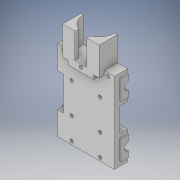
# Autodesk Inventor part: x 캐리지
Saved by Autodesk Inventor 2018 (Build 220112000, 112)
## iProperties
Created: 2019-01-22
Part Number: x 캐리지
Material: Generic
Document SubType Name: Modeling
Designer: User
Density: 1 g/cm^3
Appearance: Default
Author: User
Autodesk Inventor part; units mm, degrees
ref_plane "YZ Plane" through (0, 0, 0) normal (1, 0, 0) x (0, 1, 0)
ref_plane "XZ Plane" through (0, 0, 0) normal (0, 1, 0) x (-1, 0, 0)
ref_plane "XY Plane" through (0, 0, 0) normal (0, 0, 1) x (1, 0, 0)
sketch "스케치1" plane through (0, 0, 0) normal (1, 0, 0) x (0, 1, 0)
  arc A0 (33.25, -13) -> (18.25, -13) centre (25.75, -13) ccw
  arc A1 (-18.25, -13) -> (-33.25, -13) centre (-25.75, -13) ccw
  line L0 (-37.5, 0) -> (35.75, 0)
  line L1 (33.25, -13) -> (35.75, -13)
  line L2 (18.25, -13) -> (15.75, -13)
  line L3 (15.75, -13) -> (15.75, -5.5)
  line L4 (-18.25, -13) -> (-15.75, -13)
  line L5 (-15.75, -13) -> (-15.75, -5.5)
  line L6 (-33.25, -13) -> (-35.75, -13)
  line L7 (-35.75, -13) -> (-35.75, -5.5)
  line L8 (-15.75, -13) -> (-11.75, -13)
  line L9 (-11.75, -13) -> (-11.75, -5.5)
  line L10 (-35.75, -13) -> (-39.75, -13)
  line L11 (-39.75, -13) -> (-39.75, -5.5)
  line L12 (15.75, -13) -> (11.75, -13)
  line L13 (11.75, -13) -> (11.75, -5.5)
  line L14 (35.75, -13) -> (39.75, -13)
  line L15 (25.75, -5.5) -> (15.75, -5.5)
  line L16 (35.75, -5.5) -> (25.75, -5.5)
  line L17 (15.75, -5.5) -> (11.75, -5.5)
  line L18 (11.75, -5.5) -> (-11.75, -5.5)
  line L19 (-15.75, -5.5) -> (-25.75, -5.5)
  line L20 (-35.75, -5.5) -> (-25.75, -5.5)
  line L21 (-11.75, -5.5) -> (-15.75, -5.5)
  arc A2 (29.85, -13) -> (21.65, -13) centre (25.75, -13) ccw
  line L22 (33.25, -13) -> (29.85, -13)
  line L23 (21.65, -13) -> (18.25, -13)
  arc A3 (-21.65, -13) -> (-29.85, -13) centre (-25.75, -13) ccw
  line L24 (-18.25, -13) -> (-21.65, -13)
  line L25 (-29.85, -13) -> (-33.25, -13)
  line L26 (29.85, -13) -> (21.65, -13)
  line L27 (-21.65, -13) -> (-29.85, -13)
  line L28 (35.75, 2) -> (60.75, 2)
  line L29 (60.75, 2) -> (60.75, -13)
  line L30 (35.75, 2) -> (35.75, 0)
  line L31 (35.75, 2) -> (35.75, 5)
  line L32 (35.75, 5) -> (60.75, 5)
  line L33 (60.75, 5) -> (63.75, 5)
  line L34 (63.75, 5) -> (63.75, 2)
  line L35 (63.75, 2) -> (63.75, -13)
  line L36 (63.75, -13) -> (60.75, -13)
  line L37 (-37.5, 0) -> (-39.75, 0)
  line L38 (-39.75, 0) -> (-39.75, -5.5)
  line L39 (-35.75, -5.5) -> (-35.75, 0)
  line L40 (39.75, 0) -> (39.75, -13)
  line L41 (35.75, 0) -> (35.75, -5.5)
  line L42 (35.75, -13) -> (35.75, -5.5)
  line L43 (39.75, 0) -> (39.75, 2)
  line L44 (60.75, -13) -> (39.75, -13)
  line L45 (35.75, 5) -> (31.75, 5)
  line L46 (31.75, 5) -> (31.75, 0)
  line L47 (39.75, 0) -> (35.75, 0)
  point P0 (0, 0)
  dimension "d1" = 37.5
  dimension "d8" = 2.5
  dimension "d10" = 2.5
  dimension "d11" = 4
  dimension "d12" = 4
  dimension "d13" = 4
  dimension "d28" = 8.2
  dimension "d29" = 8.2
  dimension "d37" = 25
  dimension "d38" = 3
  dimension "d39" = 3
  dimension "d81" = 4
  constraints: 96 end point, 13 horizontal, 10 point on circle, 9 perpendicular, 9 point on line, 8 collinear, 4 centre point, 3 vertical, 2 coincident, 1 parallel, 1 tangent
  measures "d1" distance of point (0, 0) L0.start
  measures "d8" distance of L2.start L2.end
  measures "d10" distance of L6.start L6.end
  measures "d11" distance of L4.end L8.end
  measures "d12" distance of L6.end L10.end
  measures "d13" distance of L2.end L12.end
  measures "d28" diameter of A2
  measures "d29" diameter of A3
  measures "d37" distance of L28.start L28.end
  measures "d38" distance of L28.start L31.end
  measures "d39" distance of L32.end L33.end
  measures "d81" distance of L31.end L45.end
extrude "돌출1" add sketch "스케치1" along normal mid plane 56 contours L15 L17 L18 L21 L19 L20 L39 L0 L41 L16
extrude "돌출3" add sketch "스케치1" along normal mid plane 56 contours L3 L12 L13 L17 | L9 L8 L5 L21
extrude "돌출4" add sketch "스케치1" along normal mid plane 56 contours L15 L17 L18 L21 L19 L20 L39 L0 L41 L16 | L39 L7 L10 L11 L38 L37 L0
extrude "돌출5" add sketch "스케치1" along normal mid plane 52 contours A0 L16 L42 L1 | A0 L2 L3 L15 | L5 L4 A1 L19 | A1 L6 L7 L20
extrude "돌출6" add sketch "스케치1" along normal mid plane 3.8 contours L22 A2 L23 A0 | A1 L24 A3 L25
sketch "스케치3" plane through (26, 0, 0) normal (1, 0, 0) x (0, 0, -1)
  line L0 (5.5, 15.75) -> (5.5, 35.75) projected
  line L1 (13, 11.75) -> (13, 15.75) projected
  line L2 (5.5, 35.75) -> (13, 35.75)
  line L3 (13, 15.75) -> (5.5, 15.75)
  line L4 (5.5, 15.75) -> (5.5, 35.75)
  line L5 (13, 18.25) -> (13, 21.65) projected
  arc A0 (13, 29.85) -> (13, 21.65) centre (13, 25.75) ccw
  line L6 (13, 35.75) -> (13, 29.85)
  line L7 (13, 21.65) -> (13, 15.75)
  line L8 (5.5, -15.75) -> (13, -15.75) projected
  line L9 (13, -35.75) -> (13, -39.75) projected
  line L10 (5.5, -15.75) -> (13, -15.75)
  line L11 (13, -35.75) -> (5.5, -35.75)
  line L12 (5.5, -35.75) -> (5.5, -15.75)
  line L13 (13, -33.25) -> (13, -29.85) projected
  arc A1 (13, -21.65) -> (13, -29.85) centre (13, -25.75) ccw
  line L14 (13, -15.75) -> (13, -21.65)
  line L15 (13, -29.85) -> (13, -35.75)
  point P0 (0, 0)
  constraints: 21 end point, 6 parallel, 4 perpendicular, 4 point on circle, 2 centre point, 2 horizontal
extrude "돌출8" add sketch "스케치3" along normal blind 3
sketch "스케치4" plane through (-26, 0, 0) normal (-1, 0, 0) x (0, 0, 1)
  line L0 (-13, -33.25) -> (-13, -35.75) projected
  line L1 (-5.5, -15.75) -> (-13, -15.75)
  line L2 (-13, -15.75) -> (-13, -35.75)
  line L3 (-13, -35.75) -> (-5.5, -35.75)
  line L4 (-5.5, -35.75) -> (-5.5, -15.75)
  line L5 (-13, 11.75) -> (-13, 15.75) projected
  line L6 (-5.5, 35.75) -> (0, 35.75) projected
  line L7 (-13, 15.75) -> (-5.5, 15.75)
  line L8 (-5.5, 15.75) -> (-5.5, 35.75)
  line L9 (-5.5, 35.75) -> (-13, 35.75)
  arc A0 (-13, -29.85) -> (-13, -21.65) centre (-13, -25.75) ccw
  arc A1 (-13, 21.65) -> (-13, 29.85) centre (-13, 25.75) ccw
  line L10 (-13, 35.75) -> (-13, 29.85)
  line L11 (-13, 21.65) -> (-13, 15.75)
  point P0 (0, 0)
  constraints: 18 end point, 5 parallel, 4 point on circle, 2 centre point, 2 horizontal, 2 perpendicular, 2 point on line, 1 midpoint
extrude "돌출9" add sketch "스케치4" along normal blind 3 contours L2 A0 L1 L4 L3 L0 | L11 A1 L10 L9 L8 L7
extrude "돌출10" add sketch "스케치1" along normal mid plane 36 contours A0 L16 L42 L1 | L29 L28 L31 L32 L33 L34 L35 L36
sketch "스케치5" plane through (-18, 63.75, 5) normal (0, 1, 0) x (1, 0, 0)
  line L0 (0, 18) -> (36, 18) projected
  arc A0 (2.5, 18) -> (33.5, 18) centre (18, 18) ccw
  line L1 (18, 18) -> (2.5, 18)
  line L2 (-10, 18) -> (46, 18) projected
  line L3 (18, 18) -> (33.5, 18)
  line L4 (-10, 5) -> (46, 5) projected
  line L5 (23.8125, 3.6311) -> (23.8125, 0)
  line L6 (23.8125, 3.6311) -> (12.1875, 3.6311)
  line L7 (12.1875, 0) -> (23.8125, 0)
  line L8 (12.1875, 3.6311) -> (12.1875, 0)
  point P0 (18, 5)
  dimension "d43" = 31
  constraints: 12 end point, 4 point on circle, 2 point on line, 2 vertical, 1 centre point, 1 horizontal, 1 midpoint
  measures "d43" diameter of A0
sketch "스케치6" plane through (28, 11.75, -13) normal (0, 0, -1) x (-1, 0, 0)
  line L0 (28, 0) -> (28, 3.25)
  line L1 (28, 3.25) -> (14, 3.25)
  line L2 (28, 3.25) -> (42, 3.25)
  circle A0 centre (42, 3.25) radius 1.65
  circle A1 centre (14, 3.25) radius 1.65
  line L3 (28, 24.75) -> (6, 24.75)
  line L4 (28, 24.75) -> (50, 24.75)
  circle A2 centre (6, 24.75) radius 1.65
  circle A3 centre (50, 24.75) radius 1.65
  line L5 (28, 21.5) -> (28, 24.1)
  circle A4 centre (28, 24.1) radius 1.65
  line L6 (0, -23.5) -> (56, -23.5) projected
  line L7 (28, -23.5) -> (28, -26.75)
  line L8 (28, -26.75) -> (42, -26.75)
  line L9 (28, -26.75) -> (14, -26.75)
  line L10 (56, -51.5) -> (0, -51.5) projected
  line L11 (28, -51.5) -> (28, -48.25)
  line L12 (28, -48.25) -> (42, -48.25)
  line L13 (28, -48.25) -> (14, -48.25)
  circle A5 centre (14, -26.75) radius 1.65
  circle A6 centre (42, -26.75) radius 1.65
  circle A7 centre (42, -48.25) radius 1.65
  circle A8 centre (14, -48.25) radius 1.65
  point P0 (28, -11.75)
  dimension "d46" = 3.25
  dimension "d47" = 14
  dimension "d48" = 14
  dimension "d54" = 3.3
  dimension "d55" = 3.3
  dimension "d58" = 22
  dimension "d59" = 3.3
  dimension "d60" = 3.3
  dimension "d61" = 2.6
  dimension "d62" = 3.3
  dimension "d63" = 3.25
  dimension "d64" = 14
  dimension "d65" = 14
  dimension "d66" = 3.25
  dimension "d67" = 14
  dimension "d68" = 14
  dimension "d69" = 3.3
  dimension "d70" = 3.3
  dimension "d71" = 3.3
  dimension "d72" = 3.3
  constraints: 24 end point, 9 centre point, 9 coincident, 5 horizontal, 4 vertical, 3 perpendicular, 2 midpoint
  measures "d46" distance of L0.start L0.end
  measures "d47" distance of L0.end L1.end
  measures "d48" distance of L0.end L2.end
  measures "d54" diameter of A0
  measures "d55" diameter of A1
  measures "d58" distance of L3.start L4.end
  measures "d59" diameter of A2
  measures "d60" diameter of A3
  measures "d61" distance of L5.start L5.end
  measures "d62" diameter of A4
  measures "d63" distance of L7.start L7.end
  measures "d64" distance of L7.end L8.end
  measures "d65" distance of L7.end L9.end
  measures "d66" distance of L11.start L11.end
  measures "d67" distance of L11.end L12.end
  measures "d68" distance of L11.end L13.end
  measures "d69" diameter of A5
  measures "d70" diameter of A6
  measures "d71" diameter of A7
  measures "d72" diameter of A8
extrude "돌출13" add sketch "스케치1" along normal mid plane 56 contours L42 L41 L47 L40 L14 | L30 L28 L43 L47
extrude "돌출14" add sketch "스케치1" along normal mid plane 36 contours L40 L43 L28 L29 L44
extrude "돌출15" cut sketch "스케치5" against normal blind 25 contours L0 A0 L4 | L4 A0 L6 | L6 A0
extrude "돌출16" add sketch "스케치1" along normal mid plane 25 contours L0 L46 L45 L31 L30
extrude "돌출17" cut sketch "스케치6" against normal blind 20
sketch "스케치7" plane through (-28, 39.75, 2) normal (0, 0, 1) x (1, 0, 0)
  line L0 (0, -79.5) -> (0, -4) projected
  line L1 (0, 0) -> (10, 0) projected
  line L2 (0, -4) -> (10, -4)
  line L3 (10, -4) -> (10, 0)
  line L4 (10, 0) -> (0, 0)
  line L5 (0, 0) -> (0, -4)
  line L6 (46, -4) -> (46, 0) projected
  line L7 (46, -4) -> (56, -4)
  line L8 (56, -4) -> (56, 0)
  line L9 (56, 0) -> (46, 0)
  line L10 (46, 0) -> (46, -4)
  point P0 (28, -39.75)
  constraints: 16 end point, 4 parallel, 2 horizontal, 2 perpendicular
extrude "돌출18" cut sketch "스케치7" against normal blind 2
sketch "스케치8" plane through (28, 11.75, -5.5) normal (0, 0, -1) x (-1, 0, 0)
  line L0 (0, -23.5) -> (56, -23.5) projected
  line L1 (46, -23.5) -> (41, -23.5)
  line L2 (56, -23.5) -> (0, -23.5) projected
  line L3 (0, -23.5) -> (6, -23.5)
  line L4 (6, -23.5) -> (6, 0)
  line L5 (0, -23.5) -> (0, 0) projected
  line L6 (0, 0) -> (0, -23.5)
  line L7 (0, 0) -> (6, 0)
  line L8 (6, -1.75) -> (0, -1.75)
  line L9 (6, -8.25) -> (0, -8.25)
  line L10 (6, -15.25) -> (0, -15.25)
  line L11 (6, -21.75) -> (0, -21.75)
  line L12 (57, -11.75) -> (50, -11.75)
  line L13 (50, -11.75) -> (50, 4.75)
  line L14 (50, 4.75) -> (57, 4.75)
  line L15 (50, 4.75) -> (57, 4.75)
  line L16 (57, -11.75) -> (57, 4.75)
  line L17 (50, -11.75) -> (50, -28.25)
  line L18 (50, -28.25) -> (57, -28.25)
  line L19 (57, -11.75) -> (57, -28.25)
  line L20 (56, 0) -> (56, -23.5) projected
  point P0 (28, -11.75)
  dimension "d115" = 6
  dimension "d147" = 7
  dimension "d148" = 16.5
  dimension "d149" = 16.5
  constraints: 34 end point, 11 point on line, 4 perpendicular, 3 vertical, 2 collinear, 1 other
  measures "d115" distance of L0.start L3.end
  measures "d147" distance of L12.start L12.end
  measures "d148" distance of L12.end L13.end
  measures "d149" distance of L12.end L17.end
ref_plane "작업 평면3" through (28, 11.75, -13) normal (0, 0, -1) x (-1, 0, 0)
extrude "돌출28" cut sketch "스케치5" against normal blind 25 contours A0 L5 L7 L8
extrude "돌출29" cut sketch "스케치8" along normal mid plane 20 contours L17 L12 L20 L0 | L0 L20 L12 L19 L18 L17 | L13 L14 L16 L12
